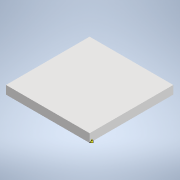
# Autodesk Inventor part: SP1848-27145 4.8V Seebeck Thermoelectric Power Generator TEG Peltier Module
Saved by Autodesk Inventor 2020 (Build 240168000, 168)
## iProperties
Created: 2021-04-27
Part Number: SP1848-27145 4.8V Seebeck Thermoelectric Power Generator TEG Peltier Module
Material: Generic
Document SubType Name: Modeling
Designer: User
Density: 1 g/cm^3
Appearance: Default
Author: User
Autodesk Inventor part; units mm, degrees
ref_plane "YZ Plane" through (0, 0, 0) normal (1, 0, 0) x (0, 1, 0)
ref_plane "XZ Plane" through (0, 0, 0) normal (0, 1, 0) x (-1, 0, 0)
ref_plane "XY Plane" through (0, 0, 0) normal (0, 0, 1) x (1, 0, 0)
sketch "Sketch1" plane through (0, 0, 0) normal (0, 1, 0) x (-1, 0, 0)
  line L0 (0, 0) -> (40, 0)
  line L1 (40, 0) -> (40, -40)
  line L2 (40, -40) -> (0, -40)
  line L3 (0, -40) -> (0, 0)
  dimension "d0" = 40
  constraints: 8 end point, 2 parallel, 2 perpendicular, 1 horizontal
  measures "d0" distance of L0.end L1.end
extrude "Extrusion1" add sketch "Sketch1" along normal blind 4
sketch "Sketch2" plane through (-40, 0, 0) normal (0, 0, 1) x (1, 0, 0)
  circle A0 centre (2, 1.9356) radius 1.4452
  line L0 (0, 0) -> (0, 4) projected
  line L1 (0, 4) -> (40, 4) projected
  line L2 (20, 17.4012) -> (20, -9.9341)
  circle A1 centre (38, 1.9356) radius 1.4452
  point P0 (40, 0)
  dimension "d3" = 2
  dimension "d4" = 40
  dimension "d5" = 20
  constraints: 2 centre point, 2 end point, 1 perpendicular, 1 symmetric about line, 1 vertical, 1 other
  measures "d3" distance from line of L0 A0.centre
  measures "d4" distance of L0.end L1.end
  measures "d5" distance between parallel lines of L0 L2
extrude "Extrusion2" add sketch "Sketch2" along normal blind 2.54
equation "\"d5\" = 0.5 * d4"
body "Solid1"
